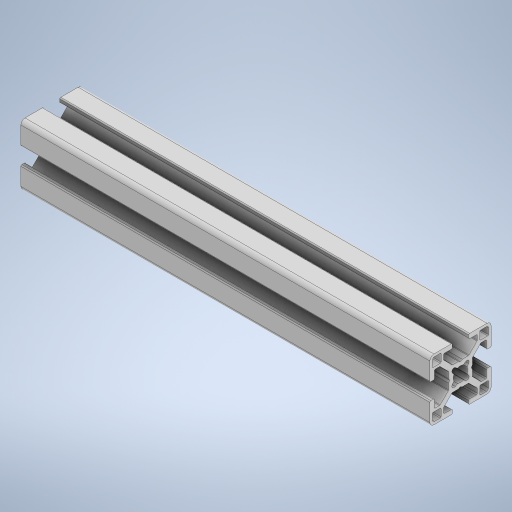
# Autodesk Inventor part: 3030_200
Saved by Autodesk Inventor 2024 (Build 280153000, 153)
## iProperties
Created: 2025-12-08
Part Number: 3030_200
Material: Generic
Document SubType Name: Modeling
Designer: schar
Density: 1 g/cm^3
Appearance: Default
Author: schar
Autodesk Inventor part; units mm, degrees
ref_plane "YZ Plane" through (0, 0, 0) normal (1, 0, 0) x (0, 1, 0)
ref_plane "XZ Plane" through (0, 0, 0) normal (0, 1, 0) x (-1, 0, 0)
ref_plane "XY Plane" through (0, 0, 0) normal (0, 0, 1) x (1, 0, 0)
sketch "Sketch1" plane through (0, 0, 0) normal (1, 0, 0) x (0, 1, 0)
  line L0 (12.6999, -13.6999) -> (9.881, -13.6999)
  arc A0 (12.6999, -13.6999) -> (13.6999, -12.6999) centre (12.6999, -12.6999) ccw
  line L1 (13.6999, -9.881) -> (13.6999, -12.6999)
  arc A1 (13.6999, -9.881) -> (13.3189, -9.5) centre (13.3189, -9.881) ccw
  line L2 (9.88, -9.5) -> (13.3189, -9.5)
  arc A2 (9.88, -9.5) -> (9.5, -9.88) centre (9.88, -9.88) ccw
  line L3 (9.5, -13.3189) -> (9.5, -9.88)
  arc A3 (9.5, -13.3189) -> (9.881, -13.6999) centre (9.881, -13.3189) ccw
  line L4 (-2.4733, 3.9799) -> (-1.4942, 3.1981)
  arc A4 (-2.4733, 3.9799) -> (-3.9799, 2.4733) centre (-3.1422, 3.1422) ccw
  line L5 (-3.1981, 1.4942) -> (-3.9799, 2.4733)
  arc A5 (-3.1981, 1.4942) -> (-3.1981, -1.4942) centre (0, 0) ccw
  line L6 (-3.9799, -2.4733) -> (-3.1981, -1.4942)
  arc A6 (-3.9799, -2.4733) -> (-2.4733, -3.9799) centre (-3.1422, -3.1422) ccw
  line L7 (-1.4942, -3.1981) -> (-2.4733, -3.9799)
  arc A7 (-1.4942, -3.1981) -> (1.4942, -3.1981) centre (0, 0) ccw
  line L8 (2.4733, -3.9799) -> (1.4942, -3.1981)
  arc A8 (2.4733, -3.9799) -> (3.9799, -2.4733) centre (3.1422, -3.1422) ccw
  line L9 (3.1981, -1.4942) -> (3.9799, -2.4733)
  arc A9 (3.1981, -1.4942) -> (3.1981, 1.4942) centre (0, 0) ccw
  line L10 (3.9799, 2.4733) -> (3.1981, 1.4942)
  arc A10 (3.9799, 2.4733) -> (2.4733, 3.9799) centre (3.1422, 3.1422) ccw
  line L11 (1.4942, 3.1981) -> (2.4733, 3.9799)
  arc A11 (1.4942, 3.1981) -> (-1.4942, 3.1981) centre (0, 0) ccw
  line L12 (9.5, 9.88) -> (9.5, 13.3189)
  arc A12 (9.5, 9.88) -> (9.88, 9.5) centre (9.88, 9.88) ccw
  line L13 (13.3189, 9.5) -> (9.88, 9.5)
  arc A13 (13.3189, 9.5) -> (13.6999, 9.881) centre (13.3189, 9.881) ccw
  line L14 (13.6999, 12.6999) -> (13.6999, 9.881)
  arc A14 (13.6999, 12.6999) -> (12.6999, 13.6999) centre (12.6999, 12.6999) ccw
  line L15 (9.881, 13.6999) -> (12.6999, 13.6999)
  arc A15 (9.881, 13.6999) -> (9.5, 13.3189) centre (9.881, 13.3189) ccw
  line L16 (12.7425, 4.5) -> (12.7425, 7.7325)
  arc A16 (12.7425, 7.7325) -> (12.2428, 8.25) centre (12.2428, 7.75) ccw
  line L17 (12.2428, 8.25) -> (10.2602, 8.25)
  arc A17 (10.2602, 8.25) -> (9.9066, 8.1035) centre (10.2602, 7.75) ccw
  line L18 (9.9066, 8.1035) -> (5.9811, 4.178)
  arc A18 (5.9811, 4.178) -> (5.8347, 3.8245) centre (6.3347, 3.8245) ccw
  line L19 (5.8347, 3.8245) -> (5.8347, 1.0125)
  line L20 (5.8347, 1.0125) -> (5.3247, 0.0625)
  line L21 (5.3247, 0.0625) -> (5.8347, -0.8875)
  line L22 (5.8347, -0.8875) -> (5.8347, -3.8245)
  arc A19 (5.8347, -3.8245) -> (5.9811, -4.178) centre (6.3347, -3.8245) ccw
  line L23 (5.9811, -4.178) -> (9.9066, -8.1035)
  arc A20 (9.9066, -8.1035) -> (10.2602, -8.25) centre (10.2602, -7.75) ccw
  line L24 (10.2602, -8.25) -> (12.2428, -8.25)
  arc A21 (12.2428, -8.25) -> (12.7425, -7.7325) centre (12.2428, -7.75) ccw
  line L25 (12.7425, -7.7325) -> (12.7425, -4.5)
  arc A22 (13.2425, -4) -> (12.7425, -4.5) centre (13.2425, -4.5) ccw
  line L26 (13.2425, -4) -> (14.4999, -4)
  arc A23 (14.9999, -4.5) -> (14.4999, -4) centre (14.4999, -4.5) ccw
  line L27 (14.9999, -4.5) -> (14.9999, -12.9999)
  arc A24 (12.9999, -14.9999) -> (14.9999, -12.9999) centre (12.9999, -12.9999) ccw
  line L28 (12.9999, -14.9999) -> (4.5, -14.9999)
  arc A25 (4, -14.4999) -> (4.5, -14.9999) centre (4.5, -14.4999) ccw
  line L29 (4, -14.4999) -> (4, -13.2425)
  arc A26 (4.5, -12.7425) -> (4, -13.2425) centre (4.5, -13.2425) ccw
  line L30 (4.5, -12.7425) -> (7.7325, -12.7425)
  arc A27 (7.7325, -12.7425) -> (8.25, -12.2428) centre (7.75, -12.2428) ccw
  line L31 (8.25, -12.2428) -> (8.25, -10.2602)
  arc A28 (8.25, -10.2602) -> (8.1035, -9.9066) centre (7.75, -10.2602) ccw
  line L32 (8.1035, -9.9066) -> (4.178, -5.9811)
  arc A29 (4.178, -5.9811) -> (3.8245, -5.8347) centre (3.8245, -6.3347) ccw
  line L33 (3.8245, -5.8347) -> (0.95, -5.8347)
  line L34 (0.95, -5.8347) -> (0, -5.3247)
  line L35 (0, -5.3247) -> (-0.95, -5.8347)
  line L36 (-0.95, -5.8347) -> (-3.8245, -5.8347)
  arc A30 (-3.8245, -5.8347) -> (-4.178, -5.9811) centre (-3.8245, -6.3347) ccw
  line L37 (-4.178, -5.9811) -> (-8.1035, -9.9066)
  arc A31 (-8.1035, -9.9066) -> (-8.25, -10.2602) centre (-7.75, -10.2602) ccw
  line L38 (-8.25, -10.2602) -> (-8.25, -12.2428)
  arc A32 (-8.25, -12.2428) -> (-7.7325, -12.7425) centre (-7.75, -12.2428) ccw
  line L39 (-7.7325, -12.7425) -> (-4.5, -12.7425)
  arc A33 (-4, -13.2425) -> (-4.5, -12.7425) centre (-4.5, -13.2425) ccw
  line L40 (-4, -13.2425) -> (-4, -14.4999)
  line L41 (-4.5, -14.9999) -> (-12.9999, -14.9999)
  arc A34 (-14.9999, -12.9999) -> (-12.9999, -14.9999) centre (-12.9999, -12.9999) ccw
  line L42 (-14.9999, -12.9999) -> (-14.9999, -4.5)
  arc A35 (-14.4999, -4) -> (-14.9999, -4.5) centre (-14.4999, -4.5) ccw
  line L43 (-14.4999, -4) -> (-13.2425, -4)
  arc A36 (-12.7425, -4.5) -> (-13.2425, -4) centre (-13.2425, -4.5) ccw
  line L44 (-12.7425, -4.5) -> (-12.7425, -7.7325)
  arc A37 (-12.7425, -7.7325) -> (-12.2428, -8.25) centre (-12.2428, -7.75) ccw
  line L45 (-12.2428, -8.25) -> (-10.2602, -8.25)
  arc A38 (-10.2602, -8.25) -> (-9.9066, -8.1035) centre (-10.2602, -7.75) ccw
  line L46 (-9.9066, -8.1035) -> (-5.9811, -4.178)
  arc A39 (-5.9811, -4.178) -> (-5.8347, -3.8245) centre (-6.3347, -3.8245) ccw
  line L47 (-5.8347, -3.8245) -> (-5.8347, -0.8875)
  line L48 (-5.8347, -0.8875) -> (-5.3247, 0.0625)
  line L49 (-5.3247, 0.0625) -> (-5.8347, 1.0125)
  line L50 (-5.8347, 1.0125) -> (-5.8347, 3.8245)
  arc A40 (-5.8347, 3.8245) -> (-5.9811, 4.178) centre (-6.3347, 3.8245) ccw
  line L51 (-5.9811, 4.178) -> (-9.9066, 8.1035)
  arc A41 (-9.9066, 8.1035) -> (-10.2602, 8.25) centre (-10.2602, 7.75) ccw
  line L52 (-10.2602, 8.25) -> (-12.2428, 8.25)
  arc A42 (-12.2428, 8.25) -> (-12.7425, 7.7325) centre (-12.2428, 7.75) ccw
  line L53 (-12.7425, 7.7325) -> (-12.7425, 4.5)
  arc A43 (-13.2425, 4) -> (-12.7425, 4.5) centre (-13.2425, 4.5) ccw
  line L54 (-13.2425, 4) -> (-14.4999, 4)
  arc A44 (-14.9999, 4.5) -> (-14.4999, 4) centre (-14.4999, 4.5) ccw
  line L55 (-14.9999, 4.5) -> (-14.9999, 12.9999)
  arc A45 (-12.9999, 14.9999) -> (-14.9999, 12.9999) centre (-12.9999, 12.9999) ccw
  line L56 (-12.9999, 14.9999) -> (-4.5, 14.9999)
  arc A46 (-4, 14.4999) -> (-4.5, 14.9999) centre (-4.5, 14.4999) ccw
  line L57 (-4, 14.4999) -> (-4, 13.2425)
  arc A47 (-4.5, 12.7425) -> (-4, 13.2425) centre (-4.5, 13.2425) ccw
  line L58 (-4.5, 12.7425) -> (-7.7325, 12.7425)
  arc A48 (-7.7325, 12.7425) -> (-8.25, 12.2428) centre (-7.75, 12.2428) ccw
  line L59 (-8.25, 12.2428) -> (-8.25, 10.2602)
  arc A49 (-8.25, 10.2602) -> (-8.1035, 9.9066) centre (-7.75, 10.2602) ccw
  line L60 (-8.1035, 9.9066) -> (-4.178, 5.9811)
  arc A50 (-4.178, 5.9811) -> (-3.8245, 5.8347) centre (-3.8245, 6.3347) ccw
  line L61 (-3.8245, 5.8347) -> (-0.95, 5.8347)
  line L62 (-0.95, 5.8347) -> (0, 5.3247)
  line L63 (0, 5.3247) -> (0.95, 5.8347)
  line L64 (0.95, 5.8347) -> (3.8245, 5.8347)
  arc A51 (3.8245, 5.8347) -> (4.178, 5.9811) centre (3.8245, 6.3347) ccw
  line L65 (4.178, 5.9811) -> (8.1035, 9.9066)
  arc A52 (8.1035, 9.9066) -> (8.25, 10.2602) centre (7.75, 10.2602) ccw
  line L66 (8.25, 10.2602) -> (8.25, 12.2428)
  arc A53 (8.25, 12.2428) -> (7.7325, 12.7425) centre (7.75, 12.2428) ccw
  line L67 (7.7325, 12.7425) -> (4.5, 12.7425)
  arc A54 (4, 13.2425) -> (4.5, 12.7425) centre (4.5, 13.2425) ccw
  line L68 (4, 13.2425) -> (4, 14.4999)
  arc A55 (4.5, 14.9999) -> (4, 14.4999) centre (4.5, 14.4999) ccw
  line L69 (4.5, 14.9999) -> (12.9999, 14.9999)
  arc A56 (14.9999, 12.9999) -> (12.9999, 14.9999) centre (12.9999, 12.9999) ccw
  line L70 (14.9999, 12.9999) -> (14.9999, 4.5)
  arc A57 (14.4999, 4) -> (14.9999, 4.5) centre (14.4999, 4.5) ccw
  line L71 (14.4999, 4) -> (13.2425, 4)
  arc A58 (12.7425, 4.5) -> (13.2425, 4) centre (13.2425, 4.5) ccw
  line L72 (-9.88, 9.5) -> (-13.3189, 9.5)
  arc A59 (-9.88, 9.5) -> (-9.5, 9.88) centre (-9.88, 9.88) ccw
  line L73 (-9.5, 13.3189) -> (-9.5, 9.88)
  arc A60 (-9.5, 13.3189) -> (-9.881, 13.6999) centre (-9.881, 13.3189) ccw
  line L74 (-12.6999, 13.6999) -> (-9.881, 13.6999)
  arc A61 (-12.6999, 13.6999) -> (-13.6999, 12.6999) centre (-12.6999, 12.6999) ccw
  line L75 (-13.6999, 9.881) -> (-13.6999, 12.6999)
  arc A62 (-13.6999, 9.881) -> (-13.3189, 9.5) centre (-13.3189, 9.881) ccw
  line L76 (-9.5, -9.88) -> (-9.5, -13.3189)
  arc A63 (-9.5, -9.88) -> (-9.88, -9.5) centre (-9.88, -9.88) ccw
  line L77 (-13.3189, -9.5) -> (-9.88, -9.5)
  arc A64 (-13.3189, -9.5) -> (-13.6999, -9.881) centre (-13.3189, -9.881) ccw
  line L78 (-13.6999, -12.6999) -> (-13.6999, -9.881)
  arc A65 (-13.6999, -12.6999) -> (-12.6999, -13.6999) centre (-12.6999, -12.6999) ccw
  line L79 (-9.881, -13.6999) -> (-12.6999, -13.6999)
  arc A66 (-9.881, -13.6999) -> (-9.5, -13.3189) centre (-9.881, -13.3189) ccw
  arc A67 (-4.5, -14.9999) -> (-4, -14.4999) centre (-4.5, -14.4999) ccw
  point P0 (14.4999, 4)
  point P1 (4, 13.2425)
  point P2 (4.178, 5.9811)
  point P3 (-3.8245, 5.8347)
  point P4 (-8.1035, 9.9066)
  point P5 (-8.25, 12.2428)
  point P6 (-4, 14.4999)
  point P7 (-12.9999, 14.9999)
  point P8 (-10.2602, 8.25)
  point P9 (-9.9066, -8.1035)
  point P10 (-14.4999, -4)
  point P11 (-14.9999, -12.9999)
  point P12 (-4, -13.2425)
  point P13 (-7.7325, -12.7425)
  point P14 (-4.178, -5.9811)
  point P15 (3.8245, -5.8347)
  point P16 (8.25, -12.2428)
  point P17 (4.5, -12.7425)
  point P18 (12.9999, -14.9999)
  point P19 (12.7425, -7.7325)
  point P20 (10.2602, -8.25)
  point P21 (5.8347, 3.8245)
  point P22 (9.9066, 8.1035)
  point P23 (12.2428, 8.25)
  point P24 (-9.88, -9.5)
  point P25 (-13.6999, -9.881)
  point P26 (-13.6999, 12.6999)
  point P27 (-9.881, 13.6999)
  point P28 (-3.9799, 2.4733)
  point P29 (2.4733, 3.9799)
  point P30 (3.1981, 1.4942)
  point P31 (3.9799, -2.4733)
  point P32 (1.4942, -3.1981)
  point P33 (-2.4733, -3.9799)
  point P34 (-3.1981, -1.4942)
  point P35 (9.5, -9.88)
  point P36 (13.3189, -9.5)
  constraints: 160 end point, 136 point on circle, 68 centre point
extrude "Extrusion1" add sketch "Sketch1" along normal blind 200
